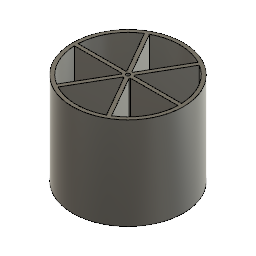
mill (Autodesk Fusion 360 design; units mm, degrees)
Autodesk Fusion 360 part; units mm, degrees
sketch "Sketch1" plane through (0, 0, 0) normal (0, 1, 0) x (1, 0, 0)
  circle A0 centre (0, 0) radius 30
  circle A1 centre (0, 0) radius 1
  circle A2 centre (0, 0) radius 2.5
  circle A3 centre (0, 0) radius 28
  dimension "d1" = 60
  dimension "d2" = 2
  dimension "d3" = 5
  dimension "d4" = 56
  measures "d1" diameter of A0
  measures "d2" diameter of A1
  measures "d3" diameter of A2
  measures "d4" diameter of A3
extrude "Extrude1" add sketch "Sketch1" along normal blind 50 makes body 1 at (29.8509, 16.6667, 2.987) makes body 2 at (2.4876, 16.6667, 0.2489)
sketch "Sketch2" plane through (0, 0, 0) normal (0, 1, 0) x (1, 0, 0)
  line L0 (-13.634, -25.6147) -> (15.366, 24.6147)
  line L1 (15.366, 24.6147) -> (13.634, 25.6147)
  line L2 (13.634, 25.6147) -> (-15.366, -24.6147)
  line L3 (-15.366, -24.6147) -> (-13.634, -25.6147)
  line L4 (-13.634, -25.6147) -> (13.634, 25.6147) construction
  line L5 (15.366, 24.6147) -> (-15.366, -24.6147) construction
  line L6 (13.634, -25.6147) -> (-15.366, 24.6147)
  line L7 (-15.366, 24.6147) -> (-13.634, 25.6147)
  line L8 (-13.634, 25.6147) -> (15.366, -24.6147)
  line L9 (15.366, -24.6147) -> (13.634, -25.6147)
  line L10 (13.634, -25.6147) -> (-13.634, 25.6147) construction
  line L11 (-15.366, 24.6147) -> (15.366, -24.6147) construction
  line L12 (29, 1) -> (-29, 1)
  line L13 (-29, 1) -> (-29, -1)
  line L14 (-29, -1) -> (29, -1)
  line L15 (29, -1) -> (29, 1)
  line L16 (29, 1) -> (-29, -1) construction
  line L17 (-29, 1) -> (29, -1) construction
  dimension "d7" = 58
  dimension "d8" = 2
  dimension "d9" = 58
  dimension "d10" = 2
  dimension "d11" = 58
  dimension "d12" = 2
extrude "Extrude2" add sketch "Sketch2" along normal blind 50 contours L0 L2 L3 L6 L14 | L0 L6 L8 L9 L14 | L2 L6 L12 L13 L14 | L0 L8 L12 L14 L15 | L0 L1 L2 L8 L12 | L2 L6 L7 L8 L12 bodies 1 2
